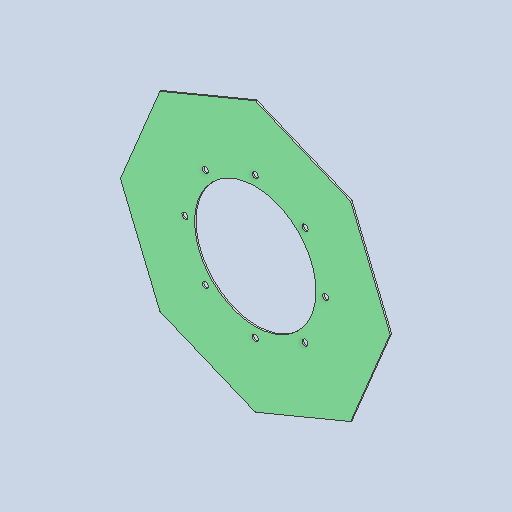
# Autodesk Inventor part: ДМФ 01 21 Барабан торец НОС v2.0
Saved by Autodesk Inventor 2025 (Build 290162010, 162A)
## iProperties
Created: 2024-04-28
Part Number: ДМФ 01 21 Барабан торец НОС v2.0
Material: Generic
Document SubType Name: Sheet Metal
Designer: pokla
Density: 1 g/cm^3
Appearance: Default
Sheet Metal Rule: Default
Flat Pattern Width: 51.3 cm
Flat Pattern Length: 51.3 cm
Flat Pattern Area: 2631.69 cm^2
Sheet Metal Width: 513,000 mm
Sheet Metal Length: 513,000 mm
Sheet Metal Area: 263169,000 mm^2
Stock Number: Барабан_Торец_Нос
Author: pokla
Autodesk Inventor part; units mm, degrees
ref_plane "YZ Plane" through (0, 0, 0) normal (1, 0, 0) x (0, 1, 0)
ref_plane "XZ Plane" through (0, 0, 0) normal (0, 1, 0) x (-1, 0, 0)
ref_plane "XY Plane" through (0, 0, 0) normal (0, 0, 1) x (1, 0, 0)
sketch "Sketch2" plane through (0, 0, 0) normal (0, 0, 1) x (1, 0, 0)
  line L0 (-196.3166, 196.3166) -> (0, 277.6336)
  line L1 (0, 277.6336) -> (196.3166, 196.3166)
  line L2 (196.3166, 196.3166) -> (277.6336, 0)
  line L3 (277.6336, 0) -> (196.3166, -196.3166)
  line L4 (196.3166, -196.3166) -> (0, -277.6336)
  line L5 (0, -277.6336) -> (-196.3166, -196.3166)
  line L6 (-196.3166, -196.3166) -> (-277.6336, 0)
  line L7 (-277.6336, 0) -> (-196.3166, 196.3166)
  circle A0 centre (0, 0) radius 125
  dimension "d23" = 513
  dimension "d26" = 250
  measures "d23" distance between parallel lines of L6 L2
  measures "d26" diameter of A0
extrude "Plate1" add sketch "Sketch2" against normal blind 3
sketch "Sketch4" plane through (0, 0, 0) normal (0, 0, 1) x (1, 0, 0)
  circle A0 centre (0, 145) radius 6.25
  circle A1 centre (0, 0) radius 125 projected
  dimension "d16" = 12.5
  dimension "d17" = 145
  constraints: 1 centre point, 1 vertical alignment
  measures "d16" diameter of A0
  measures "d17" distance of point (0, 0) A0.centre
extrude "Extrusion1" cut sketch "Sketch4" against normal up to surface (3 mm away) contours A0
pattern_circular "Circular Pattern1" count 8 over 360 about axis through (0, 0, -10) along (0, 0, 1) of "Extrusion1"
equation "\"d23\" = Барабан_габарит_по_кассетам"
equation "\"d26\" = Вал_ось_диаметр_НОС"
equation "\"d15\" = Thickness"
equation "\"BendRadius\" = Thickness"
equation "\"BendReliefWidth\" = Thickness"
equation "\"BendReliefDepth\" = 0.5 * Thickness"
equation "\"CornerReliefSize\" = 4 * Thickness"
equation "\"MinimumRemnant\" = 2 * Thickness"
equation "\"TransitionRadius\" = BendRadius"
equation "\"JacobiRadiusSize\" = BendRadius"
equation "\"GapSize\" = Thickness"
equation "\"Барабан_габарит_по_кассетам\" = 513"
equation "\"Вал_ось_диаметр_НОС\" = 250"
equation "\"Thickness\" = 3"
body "Solid1"
